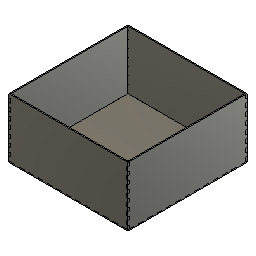
OpenField (Autodesk Fusion 360 design; units mm, degrees)
Autodesk Fusion 360 part; units mm, degrees
sketch "Floor" plane through (0, 0, 0) normal (0, 1, 0) x (1, 0, 0) in component "Main"
  line L0 (-292.1, 292.1) -> (292.1, 292.1)
  line L1 (292.1, 292.1) -> (292.1, -292.1)
  line L2 (292.1, -292.1) -> (-292.1, -292.1)
  line L3 (-292.1, -292.1) -> (-292.1, 292.1)
  line L4 (-292.1, -292.1) -> (292.1, 292.1) construction
  line L5 (-297.7, 297.7) -> (297.7, 297.7)
  line L6 (297.7, 297.7) -> (297.7, -297.7)
  line L7 (297.7, -297.7) -> (-297.7, -297.7)
  line L8 (-297.7, -297.7) -> (-297.7, 297.7)
  line L9 (0, 292.1) -> (0, 297.7) construction
  line L10 (297.7, 0) -> (292.1, 0) construction
  line L11 (-292.1, 292.1) -> (-297.7, 292.1)
  line L12 (292.1, 292.1) -> (297.7, 292.1)
  line L13 (-292.1, 292.1) -> (-292.1, 297.7)
  line L14 (-292.1, -292.1) -> (-297.7, -292.1)
  line L15 (-268.732, 292.1) -> (-268.732, 297.7)
  line L16 (-292.1, 268.732) -> (-297.7, 268.732)
  line L17 (-292.1, -292.1) -> (-292.1, -297.7)
  line L18 (-268.732, -292.1) -> (-268.732, -297.7)
  line L19 (292.1, 268.732) -> (297.7, 268.732)
  line L20 (292.1, 292.1) -> (292.1, 297.7)
  line L21 (292.1, -292.1) -> (297.7, -292.1)
  line L22 (292.1, -292.1) -> (292.1, -297.7)
  dimension "d1" = 584.2
  dimension "d3" = 5.6
  dimension "d12" = 23.368
  dimension "d13" = 23.368
  dimension "d27" = 23.368
  dimension "d28" = 23.368
  constraint horizontal L0
  constraint vertical L1
  constraint horizontal L2
  constraint vertical L3
  constraint midpoint origin L4
  constraint horizontal L5
  constraint perpendicular L2 L6
  constraint perpendicular L6 L7
  constraint perpendicular L7 L8
  constraint midpoint L0 L9.start
  constraint perpendicular L0 L9
  constraint midpoint L5 L9.end
  constraint midpoint L6 L10.start
  constraint perpendicular L1 L10
  constraint midpoint L1 L10.end
  constraint equal L9 L10
  constraint equal L0 L3
  constraint coincident L8 L11.end
  constraint perpendicular L8 L11
  constraint coincident L6 L12.end
  constraint perpendicular L6 L12
  constraint coincident L5 L13.end
  constraint perpendicular L5 L13
  constraint coincident L8 L14.end
  constraint perpendicular L8 L14
  constraint coincident L0 L15.start
  constraint coincident L5 L15.end
  constraint perpendicular L5 L15
  constraint coincident L3 L16.start
  constraint coincident L8 L16.end
  constraint perpendicular L8 L16
  constraint coincident L7 L17.end
  constraint perpendicular L7 L17
  constraint coincident L2 L18.start
  constraint coincident L7 L18.end
  constraint perpendicular L7 L18
  constraint coincident L1 L19.start
  constraint coincident L6 L19.end
  constraint perpendicular L6 L19
  constraint coincident L5 L20.end
  constraint perpendicular L5 L20
  constraint coincident L6 L21.end
  constraint perpendicular L6 L21
  constraint coincident L7 L22.end
  constraint perpendicular L7 L22
  measures "d1" distance of L0.start L0.end
  measures "d3" distance of L9.start L9.end
  measures "d12" distance of L13 L15
  measures "d13" distance of L11 L16
  measures "d27" distance of L17 L18
  measures "d28" distance of L12 L19
extrude "Extrude1" add sketch "Floor" against normal blind 5.6 contours L0 L1 L2 L3 makes body 1 in component "Main"
extrude "Extrude4" add sketch "Floor" against normal blind 5.6 contours L0 L5 L13 L15 | L2 L7 L17 L18 bodies 1 in component "Main"
pattern_linear "R-Pattern1" count 13 spacing 46.736 along (1, 0, 0) of "Extrude4" in component "Main"
extrude "Extrude5" add sketch "Floor" against normal blind 5.6 contours L3 L8 L11 L16 | L1 L6 L12 L19 bodies 1 in component "Main"
pattern_linear "R-Pattern2" count 13 spacing 46.736 along (0, 0, 1) of "Extrude5" in component "Main"
extrude "Extrude6" add sketch "Floor" against normal blind 5.6 contours L5 L8 L11 L13 | L5 L6 L12 L20 | L7 L8 L14 L17 | L6 L7 L21 L22 bodies 1 in component "Main"
extrude "Extrude2" add sketch "Floor" along normal blind 297.7 from surface at -5.6 separate body contours L0 L5 L13 L15 | L0 L5 L15 L20 makes body 2 in component "Main"
extrude "Extrude7" add sketch "Floor" along normal blind 19.4733 contours L5 L8 L11 L13 | L5 L6 L12 L20 bodies 2 in component "Main"
pattern_linear "R-Pattern3" count 8 spacing 38.9467 along (0, 1, 0) of "Extrude7" in component "Main"
combine "Combine1" operation cut target body 2 tool bodies 1 keep tools in component "Main"
mirror "Mirror1" about plane through (0, 0, 0) normal (0, 0, 1) of bodies 2 makes body 3 in component "Main"
extrude "Extrude3" add sketch "Floor" along normal blind 297.7 from surface at -5.6 separate body contours L3 L8 L11 L16 | L5 L8 L11 L13 | L3 L8 L14 L16 | L7 L8 L14 L17 makes body 4 in component "Main"
combine "Combine2" operation cut target body 4 tool bodies 2 3 1 keep tools in component "Main"
mirror "Mirror2" about plane through (0, 0, 0) normal (1, 0, 0) of bodies 4 makes body 5 in component "Main"
component "Main" placed x (1, 0, 0) y (0, 1, 0) z (0, 0, 1) at (0, 0, 0)
equation "d1 = LongL"
equation "d3 = Thick"
equation "d4 = -Thick"
equation "d6 = -Thick"
equation "d7 = ShortL + Thick"
equation "d9 = -Thick"
equation "d10 = ShortL + Thick"
equation "d12 = LongTab"
equation "d13 = LongTab"
equation "Thick = 5.6 mm"
equation "ShortL = 292.1 mm"
equation "LongL = 584.2 mm"
equation "ShortN = 15"
equation "LongN = 25"
equation "ShortTab = ShortL / ShortN"
equation "LongTab = LongL / LongN"
equation "d21 = -Thick"
equation "d23 = ( LongN + 1 ) / 2"
equation "d25 = 2 * LongTab"
equation "d27 = LongTab"
equation "d28 = LongTab"
equation "d29 = -Thick"
equation "d31 = ( LongN + 1 ) / 2"
equation "d33 = -2 * LongTab"
equation "d35 = -Thick"
equation "d37 = ShortTab"
equation "d39 = ( ShortN + 1 ) / 2"
equation "d41 = 2 * ShortTab"
named bodies: "Floor", "Side1A", "Side2A", "Side1B", "Side2B"
